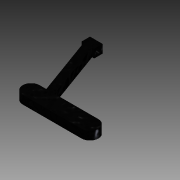
# Autodesk Inventor part: club_ABS
Saved by Autodesk Inventor 2015 SP1 (Build 190203100, 203)
## iProperties
Created: 2015-03-24
Part Number: club_ABS
Material: Ogólny
Document SubType Name: Modeling
Designer: Marcin
Density: 1 g/cm^3
Appearance: Czarny
Author: Marcin
Autodesk Inventor part; units mm, degrees
ref_plane "YZ Plane" through (0, 0, 0) normal (1, 0, 0) x (0, 1, 0)
ref_plane "XZ Plane" through (0, 0, 0) normal (0, 1, 0) x (-1, 0, 0)
ref_plane "XY Plane" through (0, 0, 0) normal (0, 0, 1) x (1, 0, 0)
sketch "Szkic1" plane through (0, 0, 0) normal (0, 0, 1) x (1, 0, 0)
  line L0 (0, 0) -> (70, 0)
  line L1 (70, 0) -> (70, 20)
  line L2 (70, 20) -> (0, 20)
  line L3 (0, 20) -> (0, 0)
  arc A0 (70, 0) -> (70, 20) centre (70, 10) ccw
  arc A1 (0, 20) -> (0, 0) centre (0, 10) ccw
  line L4 (8, 20) -> (-15.6581, 85)
  line L5 (18, 20) -> (-5.6581, 85)
  line L6 (18, 20) -> (18, 51.3428) construction
  line L7 (-5.6581, 85) -> (-15.6581, 85)
  line L8 (-18.1581, 95) -> (-3.1581, 95)
  line L9 (-3.1581, 95) -> (-3.1581, 85)
  line L10 (-3.1581, 85) -> (-18.1581, 85)
  line L11 (-18.1581, 85) -> (-18.1581, 95)
  point P0 (-10.6581, 85)
  dimension "d0" = 70
  dimension "d1" = 20
  dimension "d2" = 8
  dimension "d3" = 10
  dimension "d4" = 20
  dimension "d5" = 65
  dimension "d6" = 15
  dimension "d7" = 10
  constraints: 24 end point, 5 parallel, 4 point on circle, 3 horizontal, 2 centre point, 2 midpoint, 2 perpendicular, 2 point on line, 2 tangent, 1 vertical
  measures "d0" distance of L1.end L2.end
  measures "d1" distance of L0.end L1.end
  measures "d2" distance of L2.end L4.start
  measures "d3" distance of L5.start L4.start
  measures "d4" angle of L5 L6
  measures "d5" distance between parallel lines of L7 L2
  measures "d6" distance of L8.start L8.end
  measures "d7" distance of L8.end L9.end
extrude "Wyciągnięcie proste1" add sketch "Szkic1" along normal blind 10
sketch "Szkic2" plane through (-3.1581, 85, 0) normal (1, 0, 0) x (0, 0, -1)
  line L0 (0, 0) -> (0, 10) construction
  line L1 (0, 10) -> (-10, 10) construction
  line L2 (-10, 0) -> (-10, 10) construction
  line L3 (0, 0) -> (-10, 0) construction
  line L4 (-10, 0) -> (0, 10) construction
  point P0 (0, -85)
  point P1 (-5, 5)
  constraints: 2 end point, 1 midpoint
hole "Otwór1" at (-3.1581, 90, 5) direction (-1, 0, 0) diameter 6.35 end through all
